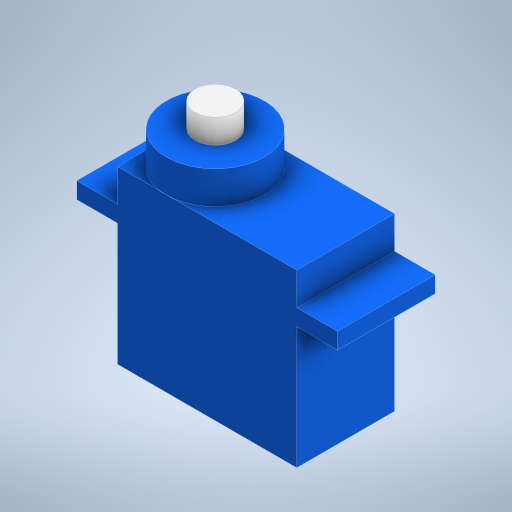
# Autodesk Inventor part: SG-90-Servo
Saved by Autodesk Inventor 2024.2 (Build 282272000, 272)
## iProperties
Created: 2024-05-04
Part Number: SG-90-Servo
Material: Generic
Document SubType Name: Modeling
Designer: ringl
Density: 1 g/cm^3
Appearance: Default(1)
Author: ringl
Autodesk Inventor part; units mm, degrees
ref_plane "YZ Plane" through (0, 0, 0) normal (1, 0, 0) x (0, 1, 0)
ref_plane "XZ Plane" through (0, 0, 0) normal (0, 1, 0) x (-1, 0, 0)
ref_plane "XY Plane" through (0, 0, 0) normal (0, 0, 1) x (1, 0, 0)
sketch "Sketch1" plane through (0, 0, 0) normal (0, 1, 0) x (-1, 0, 0)
  line L0 (0, 0) -> (22, 0)
  line L1 (22, 0) -> (22, -12)
  line L2 (22, -12) -> (0, -12)
  line L3 (0, -12) -> (0, 0)
  dimension "d0" = 22
  dimension "d1" = 12
  constraints: 8 end point, 2 parallel, 1 horizontal, 1 perpendicular
  measures "d0" distance of L1.end L2.end
  measures "d1" distance of L0.end L1.end
extrude "Extrusion1" add sketch "Sketch1" along normal blind 15
sketch "Sketch2" plane through (0, 15, 0) normal (0, 1, 0) x (1, 0, 0)
  line L0 (-27, 0) -> (5, 0)
  line L1 (5, 0) -> (5, 12)
  line L2 (5, 12) -> (-27, 12)
  line L3 (-27, 12) -> (-27, 0)
  line L4 (-22, 12) -> (-22, 0) projected
  line L5 (0, 0) -> (0, 12) projected
  point P0 (-22, 6)
  dimension "d4" = 5
  dimension "d5" = 5
  constraints: 8 end point, 2 horizontal alignment, 2 parallel, 1 horizontal, 1 midpoint, 1 perpendicular
  measures "d4" distance from line of L3 point (-22, 6)
  measures "d5" distance between parallel lines of L5 L1
extrude "Extrusion2" add sketch "Sketch2" along normal blind 2
sketch "Sketch3" plane through (0, 17, 0) normal (0, 1, 0) x (1, 0, 0)
  line L0 (-22, 0) -> (0, 0) projected
  line L1 (5, 12) -> (-27, 12) projected
  line L2 (-22, 0) -> (0, 0)
  line L3 (0, 0) -> (0, 12)
  line L4 (0, 12) -> (-22, 12)
  line L5 (-22, 12) -> (-22, 0)
  line L6 (0, 0) -> (0, 12) projected
  constraints: 8 end point, 2 parallel, 1 horizontal, 1 perpendicular
extrude "Extrusion3" add sketch "Sketch3" along normal blind 4
sketch "Sketch4" plane through (0, 21, 0) normal (0, 1, 0) x (1, 0, 0)
  circle A0 centre (-16, 6) radius 6
  line L0 (-22, 12) -> (-22, 0) projected
  line L1 (0, 12) -> (-22, 12) projected
  point P0 (0, 0)
  dimension "d10" = 12
  constraints: 2 tangent, 1 centre point
  measures "d10" diameter of A0
extrude "Extrusion4" add sketch "Sketch4" along normal blind 4 contours A0
sketch "Sketch5" plane through (-16, 25, -6) normal (0, 1, 0) x (1, 0, 0)
  circle A0 centre (0, 0) radius 2.5
  circle A1 centre (0, 0) radius 6 projected
  point P0 (16, -6)
  dimension "d13" = 5
  constraints: 1 centre point, 1 coincident
  measures "d13" diameter of A0
extrude "Extrusion5" add sketch "Sketch5" along normal blind 3 contours A0
body "Solid1"
